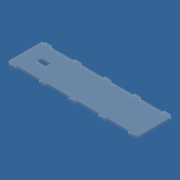
# Autodesk Inventor part: P1704_004
Saved by Autodesk Inventor 2015 (Build 190159000, 159)
## iProperties
Created: 2017-02-08
Part Number: P1704_004
Project: Manette
Material: Plastique PMMA
Description: Paroi arrière - Arcade
Document SubType Name: Modeling
Designer: Alexandre.PICOTTE
Authority: 295x83x4
Density: 1.188 g/cm^3
Appearance: Transparent - Clair
Mass: 106.795 g
Surface Area: 485.989 cm^2
Volume: 89.8949 cm^3
Material number: ---
Author: Boris.GAUDARD
Autodesk Inventor part; units mm, degrees
ref_plane "Plan YZ" through (0, 0, 0) normal (1, 0, 0) x (0, 1, 0)
ref_plane "Plan XZ" through (0, 0, 0) normal (0, 1, 0) x (-1, 0, 0)
ref_plane "Plan XY" through (0, 0, 0) normal (0, 0, 1) x (1, 0, 0)
sketch "Esquisse1" plane through (0, 0, 0) normal (0, 0, 1) x (1, 0, 0)
  line L0 (-142.5, 41.5) -> (-142.5, 37.5)
  line L1 (-142.5, 41.5) -> (-127.5, 41.5)
  line L2 (-127.5, 41.5) -> (-127.5, 37.5)
  line L3 (0, -58.1) -> (0, 58.1) construction
  line L4 (-206.5, 0) -> (206.5, 0) construction
  line L5 (-75, 41.5) -> (-75, 37.5)
  line L6 (-75, 41.5) -> (-60, 41.5)
  line L7 (-60, 41.5) -> (-60, 37.5)
  line L8 (-7.5, 41.5) -> (-7.5, 37.5)
  line L9 (-7.5, 41.5) -> (7.5, 41.5)
  line L10 (7.5, 41.5) -> (7.5, 37.5)
  line L11 (60, 41.5) -> (60, 37.5)
  line L12 (60, 41.5) -> (75, 41.5)
  line L13 (75, 41.5) -> (75, 37.5)
  line L14 (127.5, 41.5) -> (127.5, 37.5)
  line L15 (127.5, 41.5) -> (142.5, 41.5)
  line L16 (142.5, 41.5) -> (142.5, 37.5)
  line L17 (-127.5, 37.5) -> (-75, 37.5)
  line L18 (-60, 37.5) -> (-7.5, 37.5)
  line L19 (7.5, 37.5) -> (60, 37.5)
  line L20 (75, 37.5) -> (127.5, 37.5)
  line L21 (142.5, 37.5) -> (147.5, 37.5)
  line L22 (-142.5, 37.5) -> (-147.5, 37.5)
  line L23 (-142.5, -41.5) -> (-142.5, -37.5)
  line L24 (-142.5, -41.5) -> (-127.5, -41.5)
  line L25 (-127.5, -41.5) -> (-127.5, -37.5)
  line L26 (-75, -41.5) -> (-75, -37.5)
  line L27 (-75, -41.5) -> (-60, -41.5)
  line L28 (-60, -41.5) -> (-60, -37.5)
  line L29 (-7.5, -41.5) -> (-7.5, -37.5)
  line L30 (-7.5, -41.5) -> (7.5, -41.5)
  line L31 (7.5, -41.5) -> (7.5, -37.5)
  line L32 (60, -41.5) -> (60, -37.5)
  line L33 (60, -41.5) -> (75, -41.5)
  line L34 (75, -41.5) -> (75, -37.5)
  line L35 (127.5, -41.5) -> (127.5, -37.5)
  line L36 (127.5, -41.5) -> (142.5, -41.5)
  line L37 (142.5, -41.5) -> (142.5, -37.5)
  line L38 (-127.5, -37.5) -> (-75, -37.5)
  line L39 (-60, -37.5) -> (-7.5, -37.5)
  line L40 (7.5, -37.5) -> (60, -37.5)
  line L41 (75, -37.5) -> (127.5, -37.5)
  line L42 (142.5, -37.5) -> (147.5, -37.5)
  line L43 (-142.5, -37.5) -> (-147.5, -37.5)
  line L44 (147.5, -37.5) -> (147.5, 37.5)
  line L45 (-147.5, -37.5) -> (-147.5, 37.5)
  point P0 (0, 0)
  dimension "d1" = 15
  dimension "d2" = 4
  dimension "d3" = 4
  dimension "d6" = 67.5
  dimension "d11" = 5
  dimension "d12" = 5
  dimension "d30" = 75
  constraints: 88 end point, 22 symmetric about line, 3 horizontal, 2 collinear, 2 perpendicular, 2 point on line, 2 vertical, 30 other
  measures "d1" distance between parallel lines of L2 L0
  measures "d2" distance of L1.end L2.end
  measures "d3" distance of L0.start L0.end
  measures "d6" distance of L0.start L5.start
  measures "d11" distance of L0.end L22.end
  measures "d12" distance of L16.end L21.end
  measures "d30" distance between parallel lines of L22 L43
extrude "Extrusion1" add sketch "Esquisse1" along normal blind 4
sketch "Esquisse6" plane through (0, 0, 4) normal (0, 0, 1) x (1, 0, 0)
  line L0 (0, -58.1) -> (0, 58.1) construction
  line L1 (-206.5, 0) -> (206.5, 0) construction
  point P0 (0, 0)
  point P1 (-142.5, 37.5)
  point P2 (-127.5, 37.5)
  point P3 (-75, 37.5)
  point P4 (-60, 37.5)
  point P5 (-7.5, 37.5)
  point P6 (7.5, 37.5)
  point P7 (60, 37.5)
  point P8 (75, 37.5)
  point P9 (142.5, 37.5)
  point P10 (127.5, 37.5)
  point P11 (-142.5, -37.5)
  point P12 (-127.5, -37.5)
  point P13 (-75, -37.5)
  point P14 (-60, -37.5)
  point P15 (-7.5, -37.5)
  point P16 (7.5, -37.5)
  point P17 (60, -37.5)
  point P18 (75, -37.5)
  point P19 (142.5, -37.5)
  point P20 (127.5, -37.5)
  constraints: 10 symmetric about line
hole "Perçage1" at (-142.5, 37.5, 4) at (-127.5, 37.5, 4) at (-75, 37.5, 4) at (-60, 37.5, 4) at (-7.5, 37.5, 4) at (7.5, 37.5, 4) at (60, 37.5, 4) at (75, 37.5, 4) at (142.5, 37.5, 4) at (127.5, 37.5, 4) at (127.5, -37.5, 4) at (142.5, -37.5, 4) at (75, -37.5, 4) at (60, -37.5, 4) at (7.5, -37.5, 4) at (-7.5, -37.5, 4) at (-60, -37.5, 4) at (-75, -37.5, 4) at (-127.5, -37.5, 4) at (-142.5, -37.5, 4) direction (0, 0, -1) diameter 1 end through all
chamfer "Chanfrein1" distance 1 angle 45 20 edges at (-142.5, 41.5, 2) (-127.5, 41.5, 2) (-75, 41.5, 2) (-60, 41.5, 2) (-7.5, 41.5, 2) (7.5, 41.5, 2) (60, 41.5, 2) (75, 41.5, 2) (127.5, 41.5, 2) (142.5, 41.5, 2) (142.5, -41.5, 2) (127.5, -41.5, 2) (60, -41.5, 2) (75, -41.5, 2) (-142.5, -41.5, 2) (-127.5, -41.5, 2) (-75, -41.5, 2) (-60, -41.5, 2) (-7.5, -41.5, 2) (7.5, -41.5, 2)
sketch "Esquisse10" plane through (0, 0, 4) normal (0, 0, 1) x (1, 0, 0)
  line L0 (0, -58.1) -> (0, 58.1) construction
  line L1 (-206.5, 0) -> (206.5, 0) construction
  line L2 (-115, 5.5) -> (-95, 5.5)
  line L3 (-95, 5.5) -> (-95, -5.5)
  line L4 (-95, -5.5) -> (-115, -5.5)
  line L5 (-115, -5.5) -> (-115, 5.5)
  dimension "d61" = 95
  dimension "d62" = 20
  dimension "d63" = 11
  constraints: 8 end point, 2 parallel, 1 horizontal, 1 perpendicular, 1 other
  measures "d61" distance between parallel lines of L0 L3
  measures "d62" distance between parallel lines of L3 L5
  measures "d63" distance between parallel lines of L2 L4
sketch "Esquisse11" plane through (0, 0, 4) normal (0, 0, 1) x (1, 0, 0)
  line L0 (-206.5, 0) -> (206.5, 0) construction
  point P0 (0, 0)
  point P1 (-117.494, 0)
  point P2 (-92.5, 0)
  dimension "d66" = 24.994
  dimension "d69" = 92.5
  constraints: 2 point on line
  measures "d66" distance of point (-92.5, 0) point (-117.494, 0)
  measures "d69" distance of point (0, 0) point (-92.5, 0)
extrude "Extrusion4" cut sketch "Esquisse10" against normal blind 10
hole "Perçage5" at (-117.494, 0, 4) at (-92.5, 0, 4) direction (0, 0, -1) diameter 2.459 end through all thread size "M3x0.5" class "6H" standard "ISO M"
